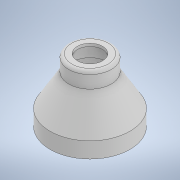
# Autodesk Inventor part: CHute2
Saved by Autodesk Inventor 2020.2 (Build 242310000, 310)
## iProperties
Created: 2020-11-09
Part Number: CHute2
Material: Generic
Document SubType Name: Modeling
Designer: JK
Density: 1 g/cm^3
Appearance: Default
Author: JK
Autodesk Inventor part; units mm, degrees
ref_plane "YZ Plane" through (0, 0, 0) normal (1, 0, 0) x (0, 1, 0)
ref_plane "XZ Plane" through (0, 0, 0) normal (0, 1, 0) x (-1, 0, 0)
ref_plane "XY Plane" through (0, 0, 0) normal (0, 0, 1) x (1, 0, 0)
sketch "Sketch1" plane through (0, 0, 0) normal (0, 1, 0) x (-1, 0, 0)
  circle A0 centre (0, 0) radius 13.5
  dimension "d0" = 27
  constraints: 1 centre point, 1 coincident
  measures "d0" diameter of A0
extrude "Extrusion1" add sketch "Sketch1" along normal blind 10
sketch "Sketch2" plane through (0, 10, 0) normal (0, 1, 0) x (1, 0, 0)
  circle A0 centre (0, 0) radius 8
  dimension "d3" = 16
  constraints: 1 centre point, 1 coincident
  measures "d3" diameter of A0
extrude "Extrusion2" cut sketch "Sketch2" against normal blind 10
chamfer "Chamfer1" distance 3 angle 70 1 edges at (-8, 0, 0) measured on face at (-8.5, 0, 0)
sketch "Sketch4" plane through (0, 0, 0) normal (1, 0, 0) x (0, 1, 0)
  line L0 (0, -13.5) -> (0, 13.5) projected
  line L1 (0, 13.5) -> (-20, 25.3)
  line L2 (0, 11) -> (0, -11) projected
  line L3 (0, 11) -> (-20, 22.8)
  line L4 (-20, 25.3) -> (-20, 22.8)
  line L5 (0, 13.5) -> (0, 11)
  line L6 (15.7921, 0) -> (-34.927, 0)
  line L7 (-20, 22.8) -> (-30, 22.8)
  line L8 (-30, 22.8) -> (-30, 25.3)
  line L9 (-30, 25.3) -> (-20, 25.3)
  line L10 (-20, 25.3) -> (-20, 22.8)
  point P0 (0, 0)
  dimension "d10" = 20
  dimension "d11" = 22.8
  dimension "d12" = 2.5
  dimension "d14" = 10
  constraints: 18 end point, 2 horizontal, 2 parallel, 2 vertical, 1 perpendicular, 1 point on line
  measures "d10" horizontal distance of L3.end point (0, 0)
  measures "d11" vertical distance of point (0, 0) L3.end
  measures "d12" distance of L3.end L1.end
  measures "d14" distance between parallel lines of L4 L8
revolve "Revolution1" add sketch "Sketch4" angle 360 about axis through (0, 15.7921, 0) along (0, -1, 0)
fillet "Fillet1" radius 2 1 edges at (13.5, 10, 0)
body "Solid1"
